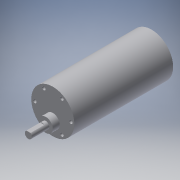
# Autodesk Inventor part: Body
Saved by Autodesk Inventor 2017 SP1 (Build 210196100, 196)
## iProperties
Created: 2017-09-02
Part Number: Body
Material: Steel, Carbon
Document SubType Name: Modeling
Designer: Zach
Density: 7.85 g/cm^3
Appearance: Default Generic
Author: Zach
Autodesk Inventor part; units mm, degrees
ref_plane "YZ Plane" through (0, 0, 0) normal (1, 0, 0) x (0, 1, 0)
ref_plane "XZ Plane" through (0, 0, 0) normal (0, 1, 0) x (-1, 0, 0)
ref_plane "XY Plane" through (0, 0, 0) normal (0, 0, 1) x (1, 0, 0)
sketch "Sketch1" plane through (0, 0, 0) normal (0, 0, 1) x (1, 0, 0)
  circle A0 centre (0, 0) radius 18.5
  dimension "d0" = 37
  constraints: 1 centre point, 1 coincident
  measures "d0" diameter of A0
extrude "Extrusion1" add sketch "Sketch1" along normal blind 85
sketch "Sketch2" plane through (0, 0, 85) normal (0, 0, 1) x (1, 0, 0)
  circle A0 centre (0, -7) radius 3
  point P0 (0, 0)
  dimension "d3" = 6
  dimension "d4" = 7
  constraints: 1 centre point, 1 vertical alignment
  measures "d3" diameter of A0
  measures "d4" distance of A0.centre point (0, 0)
extrude "Extrusion2" add sketch "Sketch2" along normal blind 21
sketch "Sketch3" plane through (0, 0, 85) normal (0, 0, 1) x (1, 0, 0)
  circle A0 centre (0, -7) radius 3 projected
  circle A1 centre (0, -7) radius 6
  point P0 (0, 0)
  dimension "d7" = 12
  constraints: 1 centre point, 1 coincident
  measures "d7" diameter of A1
extrude "Extrusion3" add sketch "Sketch3" along normal blind 6
sketch "Sketch4" plane through (0, -7, 106) normal (0, 0, 1) x (1, 0, 0)
  circle A0 centre (0, 0) radius 3 projected
  line L0 (-1.8, 2.4) -> (1.8, 2.4)
  point P0 (0, 7)
  dimension "d10" = 2.4
  constraints: 2 end point, 2 point on circle, 1 horizontal
  measures "d10" distance from line of A0.centre L0
extrude "Extrusion4" cut sketch "Sketch4" against normal blind 12 contours L0 A0 picked at (0, 2.6)
sketch "Sketch5" plane through (0, 0, 85) normal (0, 0, 1) x (1, 0, 0)
  circle A0 centre (15.5, 0) radius 1.5
  circle A1 centre (7.75, 13.4234) radius 1.5
  circle A2 centre (-7.75, 13.4234) radius 1.5
  circle A3 centre (-15.5, 0) radius 1.5
  circle A4 centre (-7.75, -13.4234) radius 1.5
  circle A5 centre (7.75, -13.4234) radius 1.5
  point P0 (0, 0)
  dimension "d13" = 3
  dimension "d14" = 15.5
  dimension "d17" = 360
  constraints: 6 centre point, 1 horizontal alignment, 13 other
  measures "d13" diameter of A0
  measures "d14" distance of A0.centre point (0, 0)
extrude "Extrusion5" cut sketch "Sketch5" against normal blind 12
body "Solid1"
